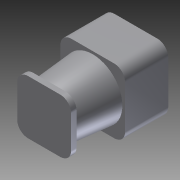
# Autodesk Inventor part: rangefinder model
Saved by Autodesk Inventor 2012 (Build 160160000, 160)
## iProperties
Created: 2011-10-07
Part Number: rangefinder model
Material: Default
Document SubType Name: Modeling
Designer: Antonella
Density: 1 g/cm^3
Author: Antonella
Autodesk Inventor part; units mm, degrees
ref_plane "YZ Plane" through (0, 0, 0) normal (1, 0, 0) x (0, 1, 0)
ref_plane "XZ Plane" through (0, 0, 0) normal (0, 1, 0) x (-1, 0, 0)
ref_plane "XY Plane" through (0, 0, 0) normal (0, 0, 1) x (1, 0, 0)
sketch "Sketch1" plane through (0, 0, 0) normal (0, 0, 1) x (1, 0, 0)
  line L0 (-53.34, 0) -> (53.34, 0) projected
  line L1 (0, -53.34) -> (0, 53.34) projected
  line L2 (-38.1, 38.1) -> (38.1, 38.1)
  line L3 (38.1, 38.1) -> (38.1, -38.1)
  line L4 (38.1, -38.1) -> (-38.1, -38.1)
  line L5 (-38.1, -38.1) -> (-38.1, 38.1)
  point P0 (0, 0)
  point P1 (-38.1, 0)
  point P2 (0, 38.1)
  dimension "d0" = 76.2
  constraints: 8 end point, 2 midpoint, 2 parallel, 2 perpendicular, 1 horizontal, 1 horizontal alignment, 1 vertical alignment
  measures "d0" distance of L4.end L2.start
extrude "Extrusion1" add sketch "Sketch1" along normal blind 50.8
sketch "Sketch2" plane through (0, 0, 50.8) normal (0, 0, 1) x (1, 0, 0)
  circle A0 centre (0, 0) radius 34.925
  dimension "d3" = 69.85
  constraints: 1 centre point, 1 coincident
  measures "d3" diameter of A0
extrude "Extrusion2" add sketch "Sketch2" along normal blind 50.8 draft -5
sketch "Sketch3" plane through (0, 0, 101.6) normal (0, 0, 1) x (1, 0, 0)
  circle A0 centre (0, 0) radius 30.4806 projected
  line L0 (-31.75, 31.75) -> (31.75, 31.75)
  line L1 (31.75, 31.75) -> (31.75, -31.75)
  line L2 (31.75, -31.75) -> (-31.75, -31.75)
  line L3 (-31.75, -31.75) -> (-31.75, 31.75)
  line L4 (-53.34, 0) -> (53.34, 0) projected
  line L5 (0, -53.34) -> (0, 53.34) projected
  point P0 (0, 31.75)
  point P1 (-31.75, 0)
  dimension "d6" = 31.75
  constraints: 8 end point, 2 midpoint, 2 parallel, 2 perpendicular, 1 horizontal, 1 horizontal alignment, 1 vertical alignment
  measures "d6" distance from line of A0.centre L0
extrude "Extrusion3" add sketch "Sketch3" along normal blind 6.35
fillet "Fillet1" radius 12.7 8 edges at (38.1, 38.1, 25.4) (38.1, -38.1, 25.4) (31.75, -31.75, 104.775) (-38.1, 38.1, 25.4) (-31.75, 31.75, 104.775) (31.75, 31.75, 104.775) (-38.1, -38.1, 25.4) (-31.75, -31.75, 104.775)
body "Solid1"
